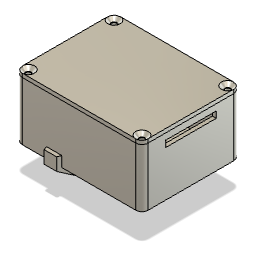
Dimmer-Box (Autodesk Fusion 360 design; units mm, degrees)
Autodesk Fusion 360 part; units mm, degrees
sketch "Sketch1" plane through (0, 0, 0) normal (0, 1, 0) x (1, 0, 0)
  line L0 (46.8, 35.75) -> (-46.8, 35.75) construction
  line L1 (-46.8, 35.75) -> (-46.8, -35.75) construction
  line L2 (-46.8, -35.75) -> (46.8, -35.75) construction
  line L3 (46.8, -35.75) -> (46.8, 35.75) construction
  line L4 (46.8, 35.75) -> (-46.8, -35.75) construction
  line L5 (-46.8, 35.75) -> (46.8, -35.75) construction
  circle A0 centre (-44.95, 33.9) radius 1.85
  line L6 (0, 0) -> (0, 35.75) construction
  line L7 (0, 0) -> (-46.8, 0) construction
  circle A1 centre (44.95, 33.9) radius 1.85
  circle A2 centre (-44.95, -33.9) radius 1.85
  circle A3 centre (44.95, -33.9) radius 1.85
  line L8 (-49.8, 38.75) -> (49.8, 38.75)
  line L9 (49.8, 38.75) -> (49.8, -38.75)
  line L10 (49.8, -38.75) -> (-49.8, -38.75)
  line L11 (-49.8, -38.75) -> (-49.8, 38.75)
  line L12 (0, 35.75) -> (0, 38.75) construction
  line L13 (-46.8, 0) -> (-49.8, 0) construction
  circle A4 centre (-44.95, 33.9) radius 4.85
  circle A5 centre (44.95, 33.9) radius 4.85
  circle A6 centre (-44.95, -33.9) radius 4.85
  circle A7 centre (44.95, -33.9) radius 4.85
  line L14 (-46.8, 29.4167) -> (-46.8, -29.4167)
  line L15 (-40.4667, -35.75) -> (40.4667, -35.75)
  line L16 (46.8, -29.4167) -> (46.8, 29.4167)
  line L17 (-40.4667, 35.75) -> (40.4667, 35.75)
  dimension "d1" = 71.5
  dimension "d2" = 93.6
  dimension "d3" = 3.7
  dimension "d4" = 3
  constraint horizontal L0
  constraint perpendicular L0 L1
  constraint parallel L0 L2
  constraint parallel L1 L3
  constraint coincident L4 L6.start
  constraint coincident L5 L6.start
  constraint coincident L6.start L7.start
  constraint tangent L0 A0
  constraint tangent L1 A0
  constraint midpoint L0 L6.end
  constraint midpoint L1 L7.end
  constraint symmetric A0 L6 A1
  constraint symmetric A0 L7 A2
  constraint symmetric L7 A1 A3
  constraint horizontal L8
  constraint vertical L9
  constraint horizontal L10
  constraint vertical L11
  constraint midpoint L8 L12.end
  constraint midpoint L11 L13.end
  constraint horizontal L13
  constraint vertical L12
  constraint equal L12 L13
  constraint concentric A0 A4
  constraint tangent L8 A4
  constraint symmetric L6 A4 A5
  constraint symmetric L7 A4 A6
  constraint symmetric L7 A5 A7
  constraint coincident A4 L14.start
  constraint coincident L1 L14.start
  constraint coincident L1 L14.end
  constraint coincident A6 L14.end
  constraint coincident A6 L15.start
  constraint coincident L2 L15.start
  constraint coincident A7 L15.end
  constraint coincident L2 L15.end
  constraint coincident A7 L16.start
  constraint coincident L3 L16.start
  constraint coincident A5 L16.end
  constraint coincident L3 L16.end
  constraint coincident A4 L17.start
  constraint coincident L0 L17.start
  constraint coincident L0 L17.end
  constraint coincident A5 L17.end
  measures "d1" distance of L0 L2
  measures "d2" distance of L1 L3
  measures "d3" diameter of A0
  measures "d4" distance of L0 L8
extrude "Extrude1" add sketch "Sketch1" along normal blind 43.05 contours L8 A4 A5 L17 | A4 | L11 A4 A6 L14 | A5 | A6 | L9 A5 A7 L16 | L10 A6 A7 L15 | A7 makes body 1
extrude "Extrude2" add sketch "Sketch1" against normal blind 3 contours A0 | A1 | A2 | A3 | L8 A4 A5 L17 | A4 | L11 A4 A6 L14 | A5 | A4 A5 A6 A7 L14 L15 L16 L17 | A6 | L9 A5 A7 L16 | L10 A6 A7 L15 | A7 bodies 1
extrude "Extrude1'" add sketch "Sketch1" along normal blind 3 from surface at 43.05 separate body contours A0 | A1 | A2 | A3 | L8 A4 A5 L17 | A4 | L11 A4 A6 L14 | A5 | A4 A5 A6 A7 L14 L15 L16 L17 | A6 | L9 A5 A7 L16 | L10 A6 A7 L15 | A7 makes body 2 in component "Lid"
sketch "Sketch3" plane through (0, 46.05, 0) normal (0, 1, 0) x (-1, 0, 0)
  line L0 (-44.95, -38.75) -> (44.95, -38.75)
  arc A0 (44.95, -38.75) -> (49.8, -33.9) centre (44.95, -33.9) ccw
  line L1 (49.8, -33.9) -> (49.8, 33.9)
  arc A1 (49.8, 33.9) -> (44.95, 38.75) centre (44.95, 33.9) ccw
  line L2 (44.95, 38.75) -> (-44.95, 38.75)
  arc A2 (-44.95, 38.75) -> (-49.8, 33.9) centre (-44.95, 33.9) ccw
  line L3 (-49.8, 33.9) -> (-49.8, -33.9)
  arc A3 (-49.8, -33.9) -> (-44.95, -38.75) centre (-44.95, -33.9) ccw
  point P0 (44.95, 33.9)
  point P1 (44.95, -33.9)
  point P2 (-44.95, -33.9)
  point P3 (-44.95, 33.9)
  constraint coincident P0 A1.centre
  constraint coincident P1 A0.centre
  constraint coincident P2 A3.centre
  constraint coincident P3 A2.centre
hole "Hole1" at (44.95, 46.05, 33.9) at (44.95, 46.05, -33.9) at (-44.95, 46.05, -33.9) at (-44.95, 46.05, 33.9) direction (0, -1, 0) diameter 4.4 depth 15 tip angle 118 countersink diameter 10 countersink angle 90 bodies 2 in component "Lid"
sketch "Sketch4" plane through (0, -3, 0) normal (0, -1, 0) x (1, 0, 0)
  arc A0 (-49.8, -33.9) -> (-44.95, -38.75) centre (-44.95, -33.9) ccw
  line L0 (-44.95, -38.75) -> (44.95, -38.75)
  arc A1 (44.95, -38.75) -> (49.8, -33.9) centre (44.95, -33.9) ccw
  line L1 (49.8, -33.9) -> (49.8, 33.9)
  arc A2 (49.8, 33.9) -> (44.95, 38.75) centre (44.95, 33.9) ccw
  line L2 (44.95, 38.75) -> (-44.95, 38.75)
  arc A3 (-44.95, 38.75) -> (-49.8, 33.9) centre (-44.95, 33.9) ccw
  line L3 (-49.8, 33.9) -> (-49.8, -33.9)
  circle A4 centre (-25.2, 0) radius 5
  line L4 (-46.8, 29.4167) -> (-46.8, -29.4167)
  dimension "d18" = 10
  dimension "d28" = 21.6
  constraint horizontal origin A4.centre
  measures "d18" diameter of A4
  measures "d28" distance of A4.centre L4
extrude "Extrude3" cut sketch "Sketch4" against normal blind 3 contours A4 bodies 1
sketch "Sketch5" plane through (49.8, 0, 0) normal (1, 0, 0) x (0, 0, -1)
  line L0 (33.9, -3) -> (33.9, 43.05)
  line L1 (33.9, 43.05) -> (-33.9, 43.05)
  line L2 (-33.9, 43.05) -> (-33.9, -3)
  line L3 (-33.9, -3) -> (33.9, -3)
  line L4 (-20, 38.05) -> (20, 38.05)
  line L5 (20, 38.05) -> (20, 33.05)
  line L6 (20, 33.05) -> (-20, 33.05)
  line L7 (-20, 33.05) -> (-20, 38.05)
  line L8 (0, 38.05) -> (0, 43.05) construction
  dimension "d30" = 40
  dimension "d31" = 5
  constraint horizontal L4
  constraint vertical L5
  constraint horizontal L6
  constraint vertical L7
  constraint midpoint L4 L8.start
  constraint midpoint L1 L8.end
  constraint equal L7 L8
  constraint vertical L8
  measures "d30" distance of L5 L7
  measures "d31" distance of L4 L6
extrude "Extrude4" cut sketch "Sketch5" against normal blind 3 contours L4 L5 L6 L7 bodies 1
sketch "Sketch6" plane through (0, 0, 0) normal (1, 0, 0) x (0, 0, -1)
  line L0 (41.75, 5.2648) -> (41.75, -4.7352)
  line L1 (41.75, -4.7352) -> (10, -23)
  line L2 (10, -23) -> (0, -23)
  line L3 (41.75, 5.2648) -> (38.75, 5.2648)
  line L4 (38.75, 5.2648) -> (38.75, -3)
  line L5 (38.75, -3) -> (9.1987, -20)
  line L6 (9.1987, -20) -> (0, -20)
  line L7 (0, -20) -> (0, -23)
  line L8 (9.1987, -20) -> (10.6946, -22.6004) construction
  point P0 (38.75, -3)
  dimension "d34" = 3
  dimension "d35" = 17
  dimension "d36" = 10
  constraint vertical L0
  constraint perpendicular L0 L2
  constraint perpendicular L0 L3
  constraint perpendicular L3 L4
  constraint perpendicular L4 L6
  constraint perpendicular L2 L7
  constraint coincident P0 L4.end
  constraint coincident origin L7
  constraint coincident L1 L8.end
  constraint perpendicular L1 L8
  constraint perpendicular L5 L8
  constraint equal L3 L8
  constraint equal L7 L8
  constraint equal L0 L2
  measures "d34" distance of L0 L4
  measures "d35" distance of P0 L6
  measures "d36" distance of L1.end L7
extrude "Extrude1''" add sketch "Sketch6" against normal blind 78 separate body makes body 3 in component "Servo Mount"
mirror "Mirror1" about plane through (0, -20, 0) normal (0, 0, 1) of bodies 3 merged in component "Servo Mount"
sketch "Sketch7" plane through (0, -23, 0) normal (0, -1, 0) x (1, 0, 0)
  line L0 (0, -10) -> (0, 10)
  line L1 (0, 10) -> (-78, 10)
  line L2 (-78, 10) -> (-78, -10)
  line L3 (-78, -10) -> (0, -10)
  circle A0 centre (-25.2, 0) radius 5 construction
  line L4 (-36.2, 10) -> (-3.2, 10)
  line L5 (-3.2, 10) -> (-3.2, -10)
  line L6 (-3.2, -10) -> (-36.2, -10)
  line L7 (-36.2, -10) -> (-36.2, 10)
  line L8 (-36.2, 10) -> (-24.7, 41.75)
  line L9 (-24.7, 41.75) -> (-14.7, 41.75)
  line L10 (-14.7, 41.75) -> (-3.2, 10)
  line L11 (-36.2, -10) -> (-24.7, -41.75)
  line L12 (-24.7, -41.75) -> (-14.7, -41.75)
  line L13 (-14.7, -41.75) -> (-3.2, -10)
  line L14 (0, -41.75) -> (-78, -41.75) construction
  line L15 (0, 41.75) -> (-78, 41.75) construction
  circle A1 centre (-34, 0) radius 1.1
  circle A2 centre (-5.4, 0) radius 1.1
  line L16 (-34, 0) -> (-5.4, 0) construction
  line L17 (-31.2, 6) -> (-8.2, 6)
  line L18 (-8.2, 6) -> (-8.2, -6)
  line L19 (-8.2, -6) -> (-31.2, -6)
  line L20 (-31.2, -6) -> (-31.2, 6)
  line L21 (-34, 0) -> (-31.2, 6) construction
  line L22 (-8.2, 6) -> (-5.4, 0) construction
  line L23 (-19.7, 0) -> (-3.2, -10) construction
  line L24 (-19.7, 0) -> (-36.2, -10) construction
  point P0 (-8.2, 0)
  point P1 (-31.2, 0)
  dimension "d43" = 10
  dimension "d46" = 2.2
  dimension "d47" = 23
  dimension "d48" = 12
  dimension "d49" = 17
  dimension "d50" = 2.8
  dimension "d51" = 33
  constraint horizontal L4
  constraint vertical L5
  constraint horizontal L6
  constraint vertical L7
  constraint coincident L3 L5.end
  constraint coincident L1 L4.start
  constraint parallel L4 L9
  constraint coincident L11.end L14
  constraint coincident L12.end L14
  constraint coincident L8.end L15
  constraint vertical L9.end L12.end
  constraint vertical L8.end L11.end
  constraint equal L8 L10
  constraint coincident A1.centre L16.start
  constraint coincident A2.centre L16.end
  constraint perpendicular L5 L16
  constraint coincident A0.centre L16
  constraint equal A1 A2
  constraint horizontal L17
  constraint vertical L18
  constraint horizontal L19
  constraint vertical L20
  constraint midpoint L18 P0
  constraint midpoint L20 P1
  constraint coincident L16 P0
  constraint equal L21 L22
  constraint midpoint L16 L23.start
  constraint equal L23 L24
  measures "d43" distance of L8.end L9.end
  measures "d46" diameter of A1
  measures "d47" distance of L18 L20
  measures "d48" distance of L17 L19
  measures "d49" distance of A0.centre L18
  measures "d50" distance of A1.centre L20
  measures "d51" distance of L5 L7
extrude "Extrude5" [suppressed]
extrude "Extrude2'" cut sketch "Sketch7" against normal up to surface (28.2648 mm away) contours L3 L6 L11 L12 L13 | L1 L3 L4 L5 L6 L7 | L1 L4 L8 L9 L10 keep common part bodies 3 in component "Servo Mount"
fillet "Fillet1" radius 40 4 edges at (-3.2, -21.2695, -10) (-3.2, -21.2695, 10) (-36.2, -21.2695, -10) (-36.2, -21.2695, 10) on bodies 3 in component "Servo Mount"
sketch "Sketch8" plane through (0, 0, 0) normal (0, 0, 1) x (1, 0, 0)
  line L0 (-20.2, -3) -> (-30.2, -3) construction
  line L1 (-25.2, -3) -> (-25.2, -23) construction
  line L2 (-3.821, -23) -> (-35.579, -23) construction
  line L3 (-20.7, -18) -> (-20.7, -10)
  line L4 (-20.7, -10) -> (-21.7, -10)
  line L5 (-21.7, -10) -> (-21.7, -13)
  line L6 (-21.7, -13) -> (-24.2, -13)
  line L7 (-24.2, -13) -> (-24.2, -14)
  line L8 (-24.2, -14) -> (-21.7, -14)
  line L9 (-21.7, -14) -> (-21.7, -18)
  line L10 (-21.7, -18) -> (-20.7, -18)
  dimension "d56" = 3.5
  dimension "d57" = 1
  dimension "d58" = 2.5
  dimension "d59" = 4
  dimension "d60" = 5
  dimension "d61" = 3
  constraint midpoint L0 L1.start
  constraint perpendicular L0 L1
  constraint coincident L1.end L2
  constraint vertical L3
  constraint perpendicular L3 L4
  constraint perpendicular L4 L5
  constraint perpendicular L1 L6
  constraint perpendicular L4 L7
  constraint perpendicular L7 L8
  constraint perpendicular L8 L9
  constraint perpendicular L3 L10
  constraint equal L4 L10
  constraint equal L7 L10
  measures "d56" distance of L1 L9
  measures "d57" distance of L3 L9
  measures "d58" distance of L5.end L6.end
  measures "d59" distance of L8 L9.end
  measures "d60" vertical distance of L1.end L9.end
  measures "d61" distance of L4 L6
revolve "Revolve1" add sketch "Sketch8" angle 360 about axis through (-25.2, -3, 0) along (0, -1, 0) separate body makes body 4 in component "Coupling"
component "Lid" placed x (1, 0, 0) y (0, 1, 0) z (0, 0, 1) at (0, 0, 0)
component "Servo Mount" placed x (1, 0, 0) y (0, 1, 0) z (0, 0, 1) at (0, 0, 0)
component "Coupling" placed x (1, 0, 0) y (0, 1, 0) z (0, 0, 1) at (0, 0, 0)
equation "d1 = box_width * 1.1"
equation "d2 = box_length * 1.2"
equation "d4 = wall_width"
equation "d6 = box_height * 1.05"
equation "d8 = -wall_width"
equation "d11 = wall_width"
equation "box_width = 65 mm" comment "The absolute width of the dimmer module"
equation "box_length = 78 mm" comment "The absolute length of the dimmer module including terminals"
equation "box_height = 41 mm" comment "The absolute height of the dimmer box, without the potentiometer"
equation "pot_hole_diameter = 10 mm" comment "The hole diameter required to house the potentiometer"
equation "wall_width = 3 mm" comment "Width of the walls of the box"
equation "d28 = pot_hole_distance * 1.2"
equation "pot_hole_distance = 18 mm" comment "The distance between the potentiometer and the top edge"
equation "d32 = -wall_width"
equation "d34 = wall_width"
equation "d37 = -box_length"
